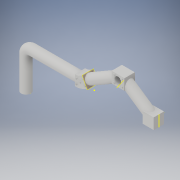
# Autodesk Inventor part: rocker (1)
Saved by Autodesk Inventor 2017 (Build 210142000, 142)
## iProperties
Created: 2017-10-20
Part Number: rocker (1)
Material: Generic
Document SubType Name: Modeling
Designer: 602199
Density: 1 g/cm^3
Appearance: Default
Author: 602199
Autodesk Inventor part; units mm, degrees
ref_plane "YZ Plane" through (0, 0, 0) normal (1, 0, 0) x (0, 1, 0)
ref_plane "XZ Plane" through (0, 0, 0) normal (0, 1, 0) x (-1, 0, 0)
ref_plane "XY Plane" through (0, 0, 0) normal (0, 0, 1) x (1, 0, 0)
sketch "Sketch1" plane through (0, 0, 0) normal (0, 1, 0) x (-1, 0, 0)
  circle A0 centre (0, 0) radius 19.05
  dimension "d0" = 38.1
  constraints: 1 centre point, 1 coincident
  measures "d0" diameter of A0
extrude "Extrusion1" add sketch "Sketch1" along normal blind 127
sketch "Sketch4" plane through (0, 127, 0) normal (0, 1, 0) x (1, 0, 0)
  circle A0 centre (0, 0) radius 19.05
  constraints: 1 centre point, 1 coincident
sketch "Sketch5" plane through (0, 0, 0) normal (0, 0, 1) x (1, 0, 0)
  line L0 (19.05, 127) -> (-19.05, 127) projected
  line L1 (-19.05, 127) -> (25.4, 127)
  arc A0 (25.4, 133.35) -> (19.05, 127) centre (25.4, 127) ccw
  arc A1 (25.4, 171.45) -> (-19.05, 127) centre (25.4, 127) ccw
  line L2 (25.4, 133.35) -> (25.4, 171.45)
  arc A2 (25.4, 152.4) -> (0, 127) centre (25.4, 127) ccw
  point P0 (0, 0)
  dimension "d6" = 44.45
  constraints: 7 point on circle, 4 end point, 3 centre point, 3 coincident, 2 point on line, 1 collinear, 1 vertical
  measures "d6" distance of L0.end L1.end
sweep "Sweep1" add profiles "Sketch4" path "Sketch5" path curves A2
sketch "Sketch6" plane through (25.4, 152.4, 0) normal (1, 0, 0) x (0, 0, -1)
  circle A0 centre (0, 0) radius 19.05
  point P0 (0, -152.4)
  constraints: 1 centre point
extrude "Extrusion2" add sketch "Sketch6" along normal blind 186.8678
sketch "Sketch7" plane through (0, 0, 0) normal (0, 0, 1) x (1, 0, 0)
  line L0 (212.2678, 133.35) -> (212.2678, 171.45) projected
  line L1 (212.2678, 171.45) -> (212.2678, 172.72)
  line L2 (224.4852, 132.08) -> (212.2678, 132.08)
  line L3 (212.2678, 132.08) -> (212.2678, 172.72)
  line L4 (212.2678, 172.72) -> (219.1258, 172.72)
  line L5 (224.4852, 132.08) -> (241.8066, 136.7212)
  line L6 (227.2142, 174.8849) -> (219.1348, 172.72)
  line L7 (224.4852, 132.08) -> (242.4176, 132.08) construction
  line L8 (241.8066, 136.7212) -> (262.0434, 146.9658)
  line L9 (262.0434, 146.9658) -> (243.6881, 183.2245)
  line L10 (243.6881, 183.2245) -> (227.2142, 174.8849)
  line L11 (223.4513, 172.9799) -> (223.5828, 172.72)
  line L12 (241.8066, 136.7212) -> (264.4888, 136.7212) construction
  line L13 (212.2678, 172.72) -> (219.1348, 172.72)
  line L14 (223.5828, 172.72) -> (224.4852, 172.72)
  point P0 (0, 0)
  dimension "d11" = 1.27
  dimension "d12" = 12.2174
  dimension "d13" = 40.64
  dimension "d14" = 6.858
  dimension "d16" = 15
  dimension "d18" = 22.6822
  dimension "d19" = 26.85
  dimension "d20" = 40.64
  constraints: 28 end point, 5 parallel, 4 horizontal, 2 equal length, 1 perpendicular, 1 point on line, 1 vertical
  measures "d11" distance of L0.end L1.end
  measures "d12" distance of L2.start L2.end
  measures "d13" distance of L14.end L2.start
  measures "d14" distance of L1.end L4.end
  measures "d16" angle of L7 L5
  measures "d18" distance of L5.end L8.end
  measures "d19" angle of L12 L8
  measures "d20" distance of L9.end L8.end
extrude "Extrusion3" add sketch "Sketch7" along normal mid plane 40.64
sketch "Sketch8" plane through (0, 0, 0) normal (0, 0, 1) x (1, 0, 0)
  line L0 (212.2678, 172.72) -> (219.1348, 172.72) projected
  line L1 (212.2678, 172.72) -> (218.0082, 172.72)
  line L2 (218.0082, 172.72) -> (218.0082, 161.9758)
  circle A0 centre (218.0082, 161.9758) radius 3.81
  line L3 (218.0082, 161.9758) -> (218.0082, 142.621) construction
  circle A1 centre (218.0082, 142.621) radius 3.81
  line L4 (218.0082, 161.9758) -> (243.6661, 172.1034) construction
  line L5 (218.0082, 161.9758) -> (245.5926, 161.9758) construction
  circle A2 centre (243.6661, 172.1034) radius 3.81
  line L6 (243.6661, 172.1034) -> (264.3925, 172.1034) construction
  circle A3 centre (252.6641, 153.4321) radius 3.81
  line L7 (218.0082, 161.9758) -> (233.313, 156.3478)
  line L8 (218.0082, 161.9758) -> (234.315, 161.9758) construction
  circle A4 centre (233.313, 156.3478) radius 3.81
  point P0 (0, 0)
  dimension "d23" = 5.7404
  dimension "d24" = 10.7442
  dimension "d25" = 7.62
  dimension "d26" = 19.3548
  dimension "d27" = 27.5844
  dimension "d28" = 21.54
  dimension "d29" = 7.62
  dimension "d32" = 7.62
  dimension "d33" = 16.3068
  dimension "d34" = 20.19
  dimension "d35" = 7.62
  constraints: 16 end point, 5 centre point, 4 coincident, 3 horizontal, 2 equal length, 1 perpendicular, 1 point on line, 1 vertical
  measures "d23" distance of L0.start L1.end
  measures "d24" distance of L1.end L2.end
  measures "d25" diameter of A0
  measures "d26" distance of L3.start L3.end
  measures "d27" distance of L3.start L4.end
  measures "d28" angle of L5 L4
  measures "d29" diameter of A2
  measures "d32" diameter of A3
  measures "d33" distance of L3.start L7.end
  measures "d34" angle of L7 L8
  measures "d35" diameter of A4
extrude "Extrusion4" add sketch "Sketch8" along normal mid plane 45.72
sketch "Sketch9" plane through (243.6881, 183.2245, 20.32) normal (0.892192, 0.4516563, 0) x (0, 0, -1)
  point P0 (20.32, -53.4081)
ref_plane "Work Plane1" through (243.6881, 183.2245, 20.32) normal (0.892192, 0.4516563, 0) x (0, 0, -1)
sketch "Sketch10" plane through (243.6881, 183.2245, 20.32) normal (0.892192, 0.4516563, 0) x (0, 0, -1)
  line L0 (40.64, -40.64) -> (0, -40.64) projected
  line L1 (20.32, -40.64) -> (20.32, -19.177)
  line L2 (20.32, -40.64) -> (41.783, -40.64) construction
  circle A0 centre (20.32, -19.177) radius 19.0754
  point P0 (20.32, -53.4081)
  dimension "d39" = 21.463
  dimension "d40" = 90
  dimension "d41" = 38.1508
  constraints: 4 end point, 1 centre point, 1 coincident, 1 horizontal, 1 midpoint, 1 perpendicular, 1 vertical
  measures "d39" distance of L1.start L1.end
  measures "d40" angle of L2 L1
  measures "d41" diameter of A0
sketch "Sketch11" plane through (0, 0, 0) normal (0, 0, 1) x (1, 0, 0)
  line L0 (252.3728, 166.1363) -> (367.1974, 232.4303)
  line L1 (252.3728, 166.1363) -> (384.9608, 166.1363) construction
  point P0 (0, 0)
  dimension "d42" = 132.588
  dimension "d43" = 30
  constraints: 4 end point, 1 equal length, 1 horizontal
  measures "d42" distance of L0.start L0.end
  measures "d43" angle of L1 L0
sweep "Sweep2" add profiles "Sketch10" path "Sketch11"
sketch "Sketch12" plane through (0, 0, 0) normal (0, 0, 1) x (1, 0, 0)
  line L0 (375.7896, 215.39) -> (358.5586, 249.4278) projected
  line L1 (358.5586, 249.4278) -> (356.4909, 248.234)
  line L2 (358.5586, 249.4278) -> (360.9462, 249.4278) construction
  line L3 (356.4909, 248.234) -> (356.4909, 256.235)
  line L4 (356.4909, 256.235) -> (407.2909, 256.235)
  line L5 (407.2909, 256.235) -> (407.2909, 213.055)
  line L6 (407.2909, 213.055) -> (356.4909, 213.055)
  line L7 (356.4909, 213.055) -> (356.4909, 256.235)
  line L8 (382.5944, 215.2082) -> (420.6182, 215.2082) construction
  point P0 (0, 0)
  dimension "d46" = 2.3876
  dimension "d47" = 150
  dimension "d48" = 8.001
  dimension "d49" = 50.8
  dimension "d50" = 43.18
  dimension "d51" = 6.8072
  constraints: 16 end point, 3 horizontal, 2 parallel, 1 equal length, 1 perpendicular, 1 vertical
  measures "d46" distance of L0.end L1.end
  measures "d47" angle of L1 L2
  measures "d48" distance of L1.end L3.end
  measures "d49" distance of L5.end L6.end
  measures "d50" distance of L4.end L5.end
  measures "d51" distance of L0.start L8.start
extrude "Extrusion5" add sketch "Sketch12" along normal mid plane 40.64
sketch "Sketch15" plane through (0, 0, 0) normal (0, 0, 1) x (1, 0, 0)
  line L0 (375.7896, 215.39) -> (358.5586, 249.4278)
  line L1 (358.5586, 249.4278) -> (360.9462, 249.4278) construction
  line L2 (382.5944, 215.2082) -> (420.6182, 215.2082) construction
  line L3 (375.7896, 215.39) -> (382.5944, 215.2082)
  line L4 (382.5944, 215.2082) -> (404.0328, 246.6122)
  line L5 (404.0328, 246.6122) -> (401.5187, 248.3285)
  line L6 (401.5187, 248.3285) -> (380.0803, 216.9246)
  line L7 (380.0803, 216.9246) -> (382.5944, 215.2082)
  line L8 (382.5944, 215.2082) -> (420.6182, 215.2082) construction
  point P0 (0, 0)
  dimension "d77" = 6.8072
  dimension "d78" = 38.0238
  dimension "d79" = 55.68
  constraints: 18 end point, 3 horizontal, 2 parallel, 1 equal length, 1 perpendicular
  measures "d77" distance of L0.start L2.start
  measures "d78" distance of L2.start L4.end
  measures "d79" angle of L8 L4
extrude "Extrusion7" add sketch "Sketch15" along normal mid plane 50.8
ref_plane "Work Plane3" through (404.0328, 246.6122, 25.4) normal (0.8259015, -0.5638144, 0) x (0, 0, -1)
sketch "Sketch16" plane through (404.0328, 246.6122, 25.4) normal (0.8259015, -0.5638144, 0) x (0, 0, -1)
  line L0 (50.8, -38.0238) -> (50.8, 0) projected
  line L1 (0, -38.0238) -> (50.8, -38.0238)
  line L2 (50.8, -38.0238) -> (50.8, 0)
  line L3 (50.8, 0) -> (0, 0)
  line L4 (0, 0) -> (0, -38.0238)
  line L5 (5.08, -38.0238) -> (45.72, -38.0238)
  line L6 (5.08, 0) -> (5.08, -38.0238)
  line L7 (45.72, 0) -> (45.72, -38.0238) projected
  line L8 (45.72, 0) -> (45.72, -38.0238)
  line L9 (5.08, -38.0238) -> (5.08, 0) projected
  line L10 (5.08, -19.0119) -> (45.72, -19.0119)
  circle A0 centre (25.4, -19.0119) radius 19.0119
  point P0 (25.4, -431.4769)
  constraints: 16 end point, 3 equal length, 3 midpoint, 2 horizontal, 1 centre point, 1 perpendicular
ref_plane "Work Plane4" through (495.2667, 138.2908, -20.32) normal (0.8259015, -0.5638144, 0) x (0, 0, -1)
sketch "Sketch17" plane through (0, 0, 0) normal (0, 0, 1) x (1, 0, 0)
  line L0 (404.0328, 246.6122) -> (382.5944, 215.2082) projected
  line L1 (393.3136, 230.9102) -> (505.9859, 153.9927)
  line L2 (393.3136, 230.9102) -> (529.737, 230.9102) construction
  point P0 (0, 0)
  dimension "d84" = 136.4234
  dimension "d85" = 34.32
  constraints: 4 end point, 1 equal length, 1 horizontal, 1 midpoint, 1 perpendicular
  measures "d84" distance of L1.start L1.end
  measures "d85" angle of L1 L2
sweep "Sweep3" add profiles "Sketch16" path "Sketch17" path curves L1 contours A0 L10 | A0 L10
sketch "Sketch18" plane through (0, 0, 25.4) normal (0, 0, 1) x (1, 0, 0)
  line L0 (401.5187, 248.3285) -> (380.0803, 216.9246) projected
  line L1 (382.5944, 215.2082) -> (404.0328, 246.6122) projected
  line L2 (380.0803, 216.9246) -> (382.5944, 215.2082)
  line L3 (382.5944, 215.2082) -> (404.0328, 246.6122)
  line L4 (404.0328, 246.6122) -> (401.5187, 248.3285)
  line L5 (401.5187, 248.3285) -> (380.0803, 216.9246)
  point P0 (0, 0)
  constraints: 8 end point, 2 parallel, 2 perpendicular
extrude "Extrusion8" cut sketch "Sketch18" against normal blind 5.08
sketch "Sketch19" plane through (0, 0, -25.4) normal (0, 0, -1) x (-1, 0, 0)
  line L0 (-382.5944, 215.2082) -> (-404.0328, 246.6122) projected
  line L1 (-401.5187, 248.3285) -> (-380.0803, 216.9246) projected
  line L2 (-404.0328, 246.6122) -> (-401.5187, 248.3285)
  line L3 (-401.5187, 248.3285) -> (-380.0803, 216.9246)
  line L4 (-380.0803, 216.9246) -> (-382.5944, 215.2082)
  line L5 (-382.5944, 215.2082) -> (-404.0328, 246.6122)
  point P0 (0, 0)
  constraints: 8 end point, 2 parallel, 2 perpendicular
extrude "Extrusion9" cut sketch "Sketch19" against normal blind 5.08
sketch "Sketch20" plane through (0, 0, 0) normal (0, 0, 1) x (1, 0, 0)
  line L0 (495.2667, 138.2908) -> (516.7051, 169.6947) projected
  line L1 (516.7051, 169.6947) -> (516.7051, 180.1595)
  line L2 (516.7051, 180.1595) -> (521.9121, 180.1595)
  line L3 (521.9121, 180.1595) -> (478.7321, 180.1595)
  line L4 (478.7321, 180.1595) -> (478.7321, 136.9795)
  line L5 (478.7321, 136.9795) -> (521.9121, 136.9795)
  line L6 (521.9121, 136.9795) -> (521.9121, 180.1595)
  point P0 (0, 0)
  dimension "d92" = 10.4648
  dimension "d93" = 5.207
  dimension "d94" = 43.18
  dimension "d95" = 43.18
  constraints: 12 end point, 2 parallel, 2 perpendicular, 1 horizontal, 1 vertical
  measures "d92" distance of L0.end L1.end
  measures "d93" distance of L1.end L2.end
  measures "d94" distance of L5.end L4.end
  measures "d95" distance of L4.end L3.end
extrude "Extrusion10" add sketch "Sketch20" along normal mid plane 40.64
sketch "Sketch21" plane through (0, 0, 0) normal (0, 0, 1) x (1, 0, 0)
  line L0 (356.4909, 213.055) -> (356.4909, 256.235) projected
  line L1 (356.4909, 256.235) -> (407.2909, 256.235) projected
  line L2 (381.2559, 256.235) -> (381.2559, 236.3214)
  circle A0 centre (381.2559, 236.3214) radius 12.7
  line L3 (356.4909, 256.235) -> (366.9303, 256.235)
  line L4 (366.9303, 256.235) -> (366.9303, 248.6658)
  circle A1 centre (366.9303, 248.6658) radius 4.4069
  line L5 (407.2909, 256.235) -> (407.2909, 213.055) projected
  line L6 (407.2909, 256.235) -> (396.8515, 256.235)
  line L7 (396.8515, 256.235) -> (396.8515, 248.6658)
  circle A2 centre (396.8515, 248.6658) radius 4.4069
  point P0 (0, 0)
  dimension "d98" = 24.765
  dimension "d99" = 19.9136
  dimension "d100" = 25.4
  dimension "d101" = 10.4394
  dimension "d102" = 7.5692
  dimension "d103" = 8.8138
  dimension "d104" = 10.4394
  dimension "d105" = 7.5692
  constraints: 10 end point, 3 centre point, 3 coincident, 3 perpendicular, 3 point on line
  measures "d98" distance of L0.end L2.start
  measures "d99" distance of L2.start L2.end
  measures "d100" diameter of A0
  measures "d101" distance of L0.end L3.end
  measures "d102" distance of L3.end L4.end
  measures "d103" diameter of A1
  measures "d104" distance of L1.end L6.end
  measures "d105" distance of L6.end L7.end
extrude "Extrusion11" cut sketch "Sketch21" along normal through all both and the other way through all contours A0
sketch "Sketch22" plane through (0, 0, 0) normal (0, 0, 1) x (1, 0, 0)
  line L0 (356.4909, 213.055) -> (356.4909, 256.235)
  line L1 (356.4909, 256.235) -> (407.2909, 256.235)
  line L2 (381.2559, 256.235) -> (381.2559, 236.3214)
  circle A0 centre (381.2559, 236.3214) radius 12.7
  line L3 (356.4909, 256.235) -> (366.9303, 256.235)
  line L4 (366.9303, 256.235) -> (366.9303, 248.6658)
  circle A1 centre (366.9303, 248.6658) radius 4.4069
  line L5 (407.2909, 256.235) -> (407.2909, 213.055)
  line L6 (407.2909, 256.235) -> (396.8515, 256.235)
  line L7 (396.8515, 256.235) -> (396.8515, 248.6658)
  circle A2 centre (396.8515, 248.6658) radius 4.4069
  line L8 (407.2909, 213.055) -> (356.4909, 213.055) projected
  line L9 (356.4909, 213.055) -> (366.9303, 213.055)
  line L10 (366.9303, 213.055) -> (366.9303, 220.802)
  circle A3 centre (366.9303, 220.802) radius 4.2418
  line L11 (407.2909, 213.055) -> (396.8515, 213.055)
  line L12 (396.8515, 213.055) -> (396.8515, 220.802)
  circle A4 centre (396.8515, 220.802) radius 4.2418
  point P0 (0, 0)
  dimension "d108" = 24.765
  dimension "d109" = 19.9136
  dimension "d110" = 25.4
  dimension "d111" = 10.4394
  dimension "d112" = 7.5692
  dimension "d113" = 8.8138
  dimension "d114" = 10.4394
  dimension "d115" = 7.5692
  dimension "d116" = 10.4394
  dimension "d117" = 7.747
  dimension "d118" = 8.4836
  dimension "d119" = 10.4394
  dimension "d120" = 8.4836
  constraints: 24 end point, 5 centre point, 5 coincident, 5 perpendicular, 5 point on line
  measures "d108" distance of L0.end L2.start
  measures "d109" distance of L2.start L2.end
  measures "d110" diameter of A0
  measures "d111" distance of L0.end L4.start
  measures "d112" distance of L4.start L4.end
  measures "d113" diameter of A1
  measures "d114" distance of L1.end L7.start
  measures "d115" distance of L7.start L7.end
  measures "d116" distance of L0.start L9.end
  measures "d117" distance of L9.end L10.end
  measures "d118" diameter of A3
  measures "d119" distance of L5.end L11.end
  measures "d120" diameter of A4
extrude "Extrusion12" add sketch "Sketch22" along normal mid plane 45.72 contours A1 | A2 | A3 | A4
sketch "Sketch23" plane through (0, 0, 0) normal (0, 0, 1) x (1, 0, 0)
  line L0 (-19.05, 0) -> (19.05, 0) projected
  line L1 (521.9121, 180.1595) -> (521.9121, 136.9795) projected
  point P0 (0, 0)
body "Solid1"
